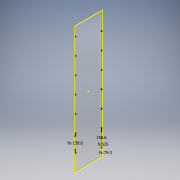
# Autodesk Inventor part: Ground_Antenna700mm_Support
Saved by Autodesk Inventor 2018 (Build 220112000, 112)
## iProperties
Created: 2018-09-26
Part Number: Ground_Antenna700mm_Support
Material: Polycarbonate, Clear
Document SubType Name: Modeling
Designer: Bradley
Mass: 1764.56 g
Surface Area: 6314.01 cm^2
Volume: 1470.47 cm^3
Density: 1.2 g/cm^3
Appearance: Polycarbonate - Clear
Author: Bradley
Autodesk Inventor part; units mm, degrees
ref_plane "YZ Plane" through (0, 0, 0) normal (1, 0, 0) x (0, 1, 0)
ref_plane "XZ Plane" through (0, 0, 0) normal (0, 1, 0) x (-1, 0, 0)
ref_plane "XY Plane" through (0, 0, 0) normal (0, 0, 1) x (1, 0, 0)
sketch "Sketch1" plane through (0, 0, 0) normal (1, 0, 0) x (0, 1, 0)
  line L0 (-130.65, -600) -> (130.65, -600)
  line L1 (130.65, -600) -> (130.65, 600)
  line L2 (130.65, 600) -> (-130.65, 600)
  line L3 (-130.65, 600) -> (-130.65, -600)
  line L4 (-130.65, -600) -> (130.65, 600) construction
  line L5 (130.65, -600) -> (-130.65, 600) construction
  line L6 (-118.65, 600) -> (-118.65, -600) construction
  line L7 (118.65, -600) -> (118.65, 600) construction
  line L8 (-118.65, 600) -> (118.65, 600) construction
  point P0 (0, 0)
  point P1 (0, 600)
  dimension "d0" = 237.3
  dimension "d1" = 12
  dimension "d2" = 1200
  constraints: 18 end point, 4 midpoint, 4 point on line, 3 perpendicular, 2 parallel, 1 collinear, 1 horizontal
  measures "d0" distance between parallel lines of L7 L6
  measures "d1" distance between parallel lines of L3 L6
  measures "d2" distance of L2.end L0.start
extrude "Extrusion1" add sketch "Sketch1" along normal mid plane 4.7625
sketch "Sketch2" plane through (2.3813, 0, 0) normal (1, 0, 0) x (0, 0, -1)
  line L0 (600, -130.65) -> (600, 130.65) projected
  line L1 (600, 130.65) -> (-600, 130.65) projected
  line L2 (-600, 130.65) -> (-600, -130.65) projected
  line L3 (-600, -130.65) -> (600, -130.65) projected
  line L4 (-600, -118.65) -> (600, -118.65) construction
  line L5 (600, 118.65) -> (-600, 118.65) construction
  circle A0 centre (520.7, 123.4125) radius 4.7625
  circle A1 centre (362.1, 123.4125) radius 4.7625
  circle A2 centre (203.5, 123.4125) radius 4.7625
  circle A3 centre (44.9, 123.4125) radius 4.7625
  circle A4 centre (-113.7, 123.4125) radius 4.7625
  circle A5 centre (-272.3, 123.4125) radius 4.7625
  circle A6 centre (-430.9, 123.4125) radius 4.7625
  circle A7 centre (441.4, -123.4125) radius 4.7625
  line L6 (362.1, 123.4125) -> (520.7, 123.4125) construction
  circle A8 centre (282.8, -123.4125) radius 4.7625
  circle A9 centre (124.2, -123.4125) radius 4.7625
  circle A10 centre (-34.4, -123.4125) radius 4.7625
  circle A11 centre (-193, -123.4125) radius 4.7625
  circle A12 centre (-351.6, -123.4125) radius 4.7625
  circle A13 centre (-510.2, -123.4125) radius 4.7625
  point P0 (0, 0)
  point P1 (441.4, 123.4125)
  dimension "d5" = 9.525
  dimension "d6" = 79.3
  dimension "d9" = 158.6
  dimension "d16" = 158.6
  constraints: 14 centre point, 2 end point, 2 horizontal, 2 tangent, 1 equal radius, 1 midpoint, 1 parallel, 1 vertical alignment, 24 other
  measures "d5" diameter of A0
  measures "d6" distance from line of L0 L6.end
  measures "d9" distance of L6.end L6.start
  measures "d16" distance of A7.centre A8.centre
equation "\"d6\" = 0.5 * d9"
equation "\"d16\" = d9"
body "Solid1"
